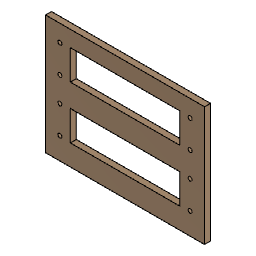
Connection box (Autodesk Fusion 360 archive; units mm, degrees)
design "Connection box socket panel"
Autodesk Fusion 360 part; units mm, degrees
sketch "Sketch1" plane through (0, 0, 0) normal (0, 1, 0) x (1, 0, 0)
  line L0 (80, -60) -> (-80, -60)
  line L1 (-80, -60) -> (-80, 60)
  line L2 (-80, 60) -> (80, 60)
  line L3 (80, 60) -> (80, -60)
  line L4 (80, -60) -> (-80, 60) construction
  line L5 (-80, -60) -> (80, 60) construction
  line L6 (0, -60) -> (0, 60) construction
  line L7 (65.5, -15) -> (-65.5, -15) construction
  line L8 (-65.5, -15) -> (-65.5, -43) construction
  line L9 (-65.5, -43) -> (65.5, -43) construction
  line L10 (65.5, -43) -> (65.5, -15) construction
  line L11 (65.5, -15) -> (-65.5, -43) construction
  line L12 (-65.5, -15) -> (65.5, -43) construction
  line L13 (65.5, 10) -> (-65.5, 10) construction
  line L14 (-65.5, 10) -> (-65.5, 38) construction
  line L15 (-65.5, 38) -> (65.5, 38) construction
  line L16 (65.5, 38) -> (65.5, 10) construction
  line L17 (65.5, 10) -> (-65.5, 38) construction
  line L18 (-65.5, 10) -> (65.5, 38) construction
  circle A0 centre (65.5, -43) radius 2
  circle A1 centre (65.5, -15) radius 2
  circle A2 centre (-65.5, -43) radius 2
  circle A3 centre (-65.5, -15) radius 2
  circle A4 centre (-65.5, 10) radius 2
  circle A5 centre (-65.5, 38) radius 2
  circle A6 centre (65.5, 38) radius 2
  circle A7 centre (65.5, 10) radius 2
  line L19 (55, -44) -> (-55, -44)
  line L20 (-55, -44) -> (-55, -14)
  line L21 (-55, -14) -> (55, -14)
  line L22 (55, -14) -> (55, -44)
  line L23 (55, -44) -> (-55, -14) construction
  line L24 (-55, -44) -> (55, -14) construction
  line L25 (55, 9) -> (-55, 9)
  line L26 (-55, 9) -> (-55, 39)
  line L27 (-55, 39) -> (55, 39)
  line L28 (55, 39) -> (55, 9)
  line L29 (55, 9) -> (-55, 39) construction
  line L30 (-55, 9) -> (55, 39) construction
  point P0 (0, -29)
  point P1 (0, 24)
  point P2 (0, -29)
  point P3 (0, 24)
  dimension "d1" = 160
  dimension "d2" = 120
  dimension "d3" = 131
  dimension "d4" = 28
  dimension "d5" = 131
  dimension "d6" = 28
  dimension "d7" = 15
  dimension "d8" = 10
  dimension "d9" = 4
  dimension "d10" = 4
  dimension "d11" = 4
  dimension "d12" = 4
  dimension "d13" = 4
  dimension "d14" = 4
  dimension "d15" = 4
  dimension "d16" = 4
  dimension "d17" = 110
  dimension "d18" = 30
  dimension "d19" = 110
  dimension "d20" = 30
  constraint perpendicular L0 L1
  constraint parallel L0 L2
  constraint parallel L1 L3
  constraint horizontal L0
  constraint coincident L4 origin
  constraint coincident L5 origin
  constraint midpoint L0 L6.start
  constraint midpoint L2 L6.end
  constraint perpendicular L7 L8
  constraint parallel L7 L9
  constraint parallel L8 L10
  constraint horizontal L7
  constraint coincident L11 P2
  constraint coincident L12 P2
  constraint coincident L6 P2
  constraint perpendicular L13 L14
  constraint parallel L13 L15
  constraint parallel L14 L16
  constraint horizontal L13
  constraint coincident L17 P3
  constraint coincident L18 P3
  constraint coincident L6 P3
  constraint coincident L9.end L10.start
  constraint coincident L7.start L10.end
  constraint coincident L8.end L9.start
  constraint coincident L7.end L8.start
  constraint coincident L13.end L14.start
  constraint coincident L14.end L15.start
  constraint coincident L15.end L16.start
  constraint coincident L13.start L16.end
  constraint perpendicular L19 L20
  constraint parallel L19 L21
  constraint parallel L20 L22
  constraint horizontal L19
  constraint coincident L23 P2
  constraint coincident L24 P2
  constraint coincident P2 P0
  constraint perpendicular L25 L26
  constraint parallel L25 L27
  constraint parallel L26 L28
  constraint horizontal L25
  constraint coincident L29 P3
  constraint coincident L30 P3
  constraint coincident P3 P1
  measures "d1" distance of L1.end L2.end
  measures "d2" distance of L0.end L1.end
  measures "d3" distance of L8.end L9.end
  measures "d4" distance of L7.end L8.end
  measures "d5" distance of L14.end L15.end
  measures "d6" distance of L13.end L14.end
  measures "d7" distance of origin L7
  measures "d8" distance of origin L13
  measures "d9" diameter of A0
  measures "d10" diameter of A1
  measures "d11" diameter of A2
  measures "d12" diameter of A3
  measures "d13" diameter of A4
  measures "d14" diameter of A5
  measures "d15" diameter of A6
  measures "d16" diameter of A7
  measures "d17" distance of L20.end L21.end
  measures "d18" distance of L19.end L20.end
  measures "d19" distance of L26.end L27.end
  measures "d20" distance of L25.end L26.end
extrude "Extrude2" add sketch "Sketch1" along normal blind 6
extrude "Extrude1" [suppressed]
equation "d3 = 143 mm - 12 mm"
equation "d4 = 40 mm - 12 mm"
equation "d5 = 143 mm - 12 mm"
equation "d6 = 40 mm - 12 mm"
equation "d10 = d9"
equation "d11 = d9"
equation "d12 = d9"
equation "d13 = d9"
equation "d14 = d9"
equation "d15 = d9"
equation "d16 = d9"
named bodies: "Panel"

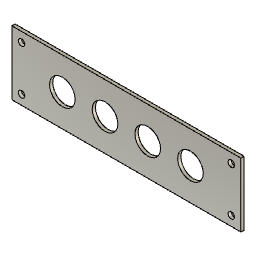
design "4 hole plate"
Autodesk Fusion 360 part; units mm, degrees
sketch "Sketch1" plane through (0, 0, 0) normal (0, 1, 0) x (1, 0, 0)
  line L0 (0, 0) -> (0, -50.0731) construction
  line L1 (-71.5, 0) -> (71.5, 0)
  line L2 (71.5, 0) -> (71.5, -40)
  line L3 (71.5, -40) -> (-71.5, -40)
  line L4 (-71.5, -40) -> (-71.5, 0)
  line L5 (-71.5, -20) -> (71.5, -20) construction
  line L6 (-65.5, -34) -> (65.5, -34) construction
  line L7 (65.5, -34) -> (65.5, -6) construction
  line L8 (65.5, -6) -> (-65.5, -6) construction
  line L9 (-65.5, -6) -> (-65.5, -34) construction
  circle A0 centre (-65.5, -34) radius 2
  circle A1 centre (65.5, -34) radius 2
  circle A2 centre (65.5, -6) radius 2
  circle A3 centre (-65.5, -6) radius 2
  circle A4 centre (13.3333, -20) radius 8
  circle A5 centre (40, -20) radius 8
  circle A6 centre (-13.3333, -20) radius 8
  circle A7 centre (-40, -20) radius 8
  dimension "d1" = 143
  dimension "d2" = 40
  dimension "d3" = 71.5
  dimension "d4" = 40
  dimension "d5" = 6
  dimension "d6" = 6
  dimension "d7" = 6
  dimension "d8" = 6
  dimension "d9" = 4
  dimension "d10" = 4
  dimension "d11" = 4
  dimension "d12" = 4
  dimension "d15" = 16
  dimension "d16" = 16
  dimension "d17" = 16
  dimension "d18" = 16
  dimension "d19" = 26.6667
  dimension "d20" = 26.6667
  dimension "d21" = 26.6667
  dimension "d22" = 13.3333
  constraint coincident L0.start origin
  constraint vertical L0
  constraint horizontal L1
  constraint vertical L2
  constraint horizontal L3
  constraint vertical L4
  constraint midpoint L4 L5.start
  constraint midpoint L2 L5.end
  constraint horizontal L6
  constraint vertical L7
  constraint horizontal L8
  constraint vertical L9
  constraint coincident L6.start L9.end
  constraint coincident L6.end L7.start
  constraint coincident L7.end L8.start
  constraint coincident L8.end L9.start
  constraint coincident L5 A4.centre
  constraint coincident L5 A5.centre
  constraint coincident L5 A6.centre
  constraint coincident L5 A7.centre
  measures "d1" distance of L1.start L1.end
  measures "d2" distance of L1.start L3.end
  measures "d3" distance of L0 L2
  measures "d4" distance of L0.start L3
  measures "d5" distance of L3 L6
  measures "d6" distance of L1 L8
  measures "d7" distance of L2 L7
  measures "d8" distance of L4 L9
  measures "d9" diameter of A0
  measures "d10" diameter of A1
  measures "d11" diameter of A2
  measures "d12" diameter of A3
  measures "d15" diameter of A4
  measures "d16" diameter of A5
  measures "d17" diameter of A6
  measures "d18" diameter of A7
  measures "d19" distance of A6.centre A7.centre
  measures "d20" distance of A4.centre A6.centre
  measures "d21" distance of A4.centre A5.centre
  measures "d22" distance of L0 A4.centre
extrude "Extrude1" add sketch "Sketch1" along normal blind 2
equation "d3 = d1 / 2"
equation "d4 = d2"
equation "d6 = d5"
equation "d8 = d7"
equation "d10 = d9"
equation "d11 = d9"
equation "d12 = d9"
equation "HoleSpread = 80 mm"
equation "HoleDia = 16 mm"
equation "d15 = HoleDia"
equation "d16 = HoleDia"
equation "d17 = HoleDia"
equation "d18 = HoleDia"
equation "d19 = HoleSpread / 3"
equation "d20 = HoleSpread / 3"
equation "d21 = HoleSpread / 3"
equation "d22 = HoleSpread / 6"
named bodies: "Panel"

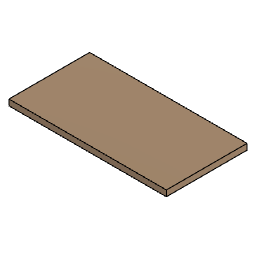
design "Connection box lid"
Autodesk Fusion 360 part; units mm, degrees
sketch "Sketch1" plane through (0, 0, 0) normal (0, 0, 1) x (1, 0, 0)
  line L0 (74, -35) -> (-74, -35)
  line L1 (-74, -35) -> (-74, 35)
  line L2 (-74, 35) -> (74, 35)
  line L3 (74, 35) -> (74, -35)
  line L4 (74, -35) -> (-74, 35) construction
  line L5 (-74, -35) -> (74, 35) construction
  line L6 (80, 41) -> (-80, 41)
  line L7 (-80, 41) -> (-80, -41)
  line L8 (-80, -41) -> (80, -41)
  line L9 (80, -41) -> (80, 41)
  line L10 (80, 41) -> (-80, -41) construction
  line L11 (-80, 41) -> (80, -41) construction
  dimension "d1" = 148
  dimension "d2" = 70
  dimension "d3" = 160
  dimension "d4" = 82
  constraint perpendicular L0 L1
  constraint parallel L0 L2
  constraint parallel L1 L3
  constraint horizontal L0
  constraint coincident L4 origin
  constraint coincident L5 origin
  constraint perpendicular L6 L7
  constraint parallel L6 L8
  constraint parallel L7 L9
  constraint horizontal L6
  constraint coincident L10 origin
  constraint coincident L11 origin
  measures "d1" distance of L1.end L2.end
  measures "d2" distance of L0.end L1.end
  measures "d3" distance of L7.end L8.end
  measures "d4" distance of L6.end L7.end
extrude "Extrude1" add sketch "Sketch1" against normal blind 6 contours L0 L1 L2 L3 makes body 1
extrude "Extrude2" add sketch "Sketch1" along normal blind 6 separate body contours L0 L1 L2 L3 | L6 L7 L8 L9 makes body 2
equation "d3 = d1 + 12 mm"
equation "d4 = d2 + 12 mm"
named bodies: "Inset", "Lid"

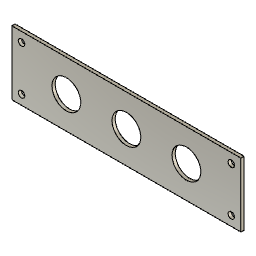
design "3 hole plate"
Autodesk Fusion 360 part; units mm, degrees
sketch "Sketch1" plane through (0, 0, 0) normal (0, 1, 0) x (1, 0, 0)
  line L0 (0, 0) -> (0, -50.0731) construction
  line L1 (-71.5, 0) -> (71.5, 0)
  line L2 (71.5, 0) -> (71.5, -40)
  line L3 (71.5, -40) -> (-71.5, -40)
  line L4 (-71.5, -40) -> (-71.5, 0)
  line L5 (-71.5, -20) -> (71.5, -20) construction
  line L6 (-65.5, -34) -> (65.5, -34) construction
  line L7 (65.5, -34) -> (65.5, -6) construction
  line L8 (65.5, -6) -> (-65.5, -6) construction
  line L9 (-65.5, -6) -> (-65.5, -34) construction
  circle A0 centre (-65.5, -34) radius 2
  circle A1 centre (65.5, -34) radius 2
  circle A2 centre (65.5, -6) radius 2
  circle A3 centre (-65.5, -6) radius 2
  circle A4 centre (37.5, -20) radius 9
  circle A5 centre (-37.5, -20) radius 9
  circle A6 centre (0, -20) radius 9
  dimension "d1" = 143
  dimension "d2" = 40
  dimension "d3" = 71.5
  dimension "d4" = 40
  dimension "d5" = 6
  dimension "d6" = 6
  dimension "d7" = 6
  dimension "d8" = 6
  dimension "d9" = 4
  dimension "d10" = 4
  dimension "d11" = 4
  dimension "d12" = 4
  dimension "d16" = 18
  dimension "d17" = 18
  dimension "d25" = 18
  dimension "d26" = 37.5
  dimension "d27" = 37.5
  constraint coincident L0.start origin
  constraint vertical L0
  constraint horizontal L1
  constraint vertical L2
  constraint horizontal L3
  constraint vertical L4
  constraint midpoint L4 L5.start
  constraint midpoint L2 L5.end
  constraint horizontal L6
  constraint vertical L7
  constraint horizontal L8
  constraint vertical L9
  constraint coincident L6.start L9.end
  constraint coincident L6.end L7.start
  constraint coincident L7.end L8.start
  constraint coincident L8.end L9.start
  constraint coincident L5 A4.centre
  constraint coincident L5 A5.centre
  constraint midpoint L5 A6.centre
  measures "d1" distance of L1.start L1.end
  measures "d2" distance of L1.start L3.end
  measures "d3" distance of L0 L2
  measures "d4" distance of L0.start L3
  measures "d5" distance of L3 L6
  measures "d6" distance of L1 L8
  measures "d7" distance of L2 L7
  measures "d8" distance of L4 L9
  measures "d9" diameter of A0
  measures "d10" diameter of A1
  measures "d11" diameter of A2
  measures "d12" diameter of A3
  measures "d16" diameter of A4
  measures "d17" diameter of A5
  measures "d25" diameter of A6
  measures "d26" distance of A5.centre A6.centre
  measures "d27" distance of A4.centre A6.centre
extrude "Extrude1" add sketch "Sketch1" along normal blind 2
equation "d3 = d1 / 2"
equation "d4 = d2"
equation "d6 = d5"
equation "d8 = d7"
equation "d10 = d9"
equation "d11 = d9"
equation "d12 = d9"
equation "HoleSpread = 75 mm"
equation "HoleDia = 18 mm"
equation "d16 = HoleDia"
equation "d17 = HoleDia"
equation "d25 = HoleDia"
equation "d26 = HoleSpread / 2"
equation "d27 = HoleSpread / 2"
named bodies: "Panel"

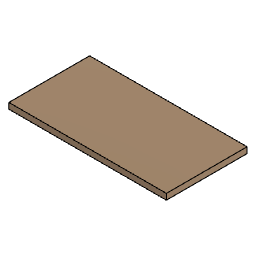
design "Connection box top"
Autodesk Fusion 360 part; units mm, degrees
sketch "Sketch1" plane through (0, 0, 0) normal (0, 0, 1) x (1, 0, 0)
  line L0 (80, -41) -> (-80, -41)
  line L1 (-80, -41) -> (-80, 41)
  line L2 (-80, 41) -> (80, 41)
  line L3 (80, 41) -> (80, -41)
  line L4 (80, -41) -> (-80, 41) construction
  line L5 (-80, -41) -> (80, 41) construction
  dimension "d1" = 160
  dimension "d2" = 82
  constraint perpendicular L0 L1
  constraint parallel L0 L2
  constraint parallel L1 L3
  constraint horizontal L0
  constraint coincident L4 origin
  constraint coincident L5 origin
  measures "d1" distance of L1.end L2.end
  measures "d2" distance of L0.end L1.end
extrude "Extrude1" add sketch "Sketch1" along normal blind 6
named bodies: "Panel"

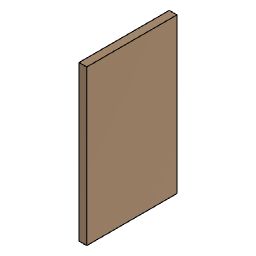
design "Connection box side panel"
Autodesk Fusion 360 part; units mm, degrees
sketch "Sketch1" plane through (0, 0, 0) normal (1, 0, 0) x (0, 1, 0)
  line L0 (35, 60) -> (-35, 60)
  line L1 (-35, 60) -> (-35, -60)
  line L2 (-35, -60) -> (35, -60)
  line L3 (35, -60) -> (35, 60)
  line L4 (35, 60) -> (-35, -60) construction
  line L5 (-35, 60) -> (35, -60) construction
  dimension "d1" = 70
  dimension "d2" = 120
  constraint perpendicular L0 L1
  constraint parallel L0 L2
  constraint parallel L1 L3
  constraint horizontal L0
  constraint coincident L4 origin
  constraint coincident L5 origin
  measures "d1" distance of L1.end L2.end
  measures "d2" distance of L0.end L1.end
extrude "Extrude1" add sketch "Sketch1" along normal blind 6
named bodies: "Panel"

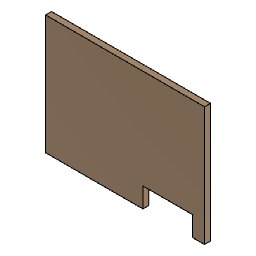
design "Connection box rear panel"
Autodesk Fusion 360 part; units mm, degrees
sketch "Sketch1" plane through (0, 0, 0) normal (0, 1, 0) x (1, 0, 0)
  line L0 (80, -60) -> (-80, -60)
  line L1 (-80, -60) -> (-80, 60)
  line L2 (-80, 60) -> (80, 60)
  line L3 (80, 60) -> (80, -60)
  line L4 (80, -60) -> (-80, 60) construction
  line L5 (-80, -60) -> (80, 60) construction
  line L6 (18, 60) -> (68, 60)
  line L7 (68, 60) -> (68, 40)
  line L8 (68, 40) -> (18, 40)
  line L9 (18, 40) -> (18, 60)
  dimension "d1" = 160
  dimension "d2" = 120
  dimension "d3" = 50
  dimension "d4" = 20
  dimension "d5" = 12
  constraint perpendicular L0 L1
  constraint parallel L0 L2
  constraint parallel L1 L3
  constraint horizontal L0
  constraint coincident L4 origin
  constraint coincident L5 origin
  constraint horizontal L6
  constraint vertical L7
  constraint horizontal L8
  constraint vertical L9
  constraint coincident L2 L6.start
  measures "d1" distance of L1.end L2.end
  measures "d2" distance of L0.end L1.end
  measures "d3" distance of L6.start L6.end
  measures "d4" distance of L6.start L8.end
  measures "d5" distance of L3 L7
extrude "Extrude1" add sketch "Sketch1" along normal blind 6 contours L0 L1 L2 L3 L7 L8 L9
named bodies: "Panel"
